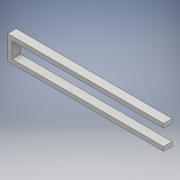
# Autodesk Inventor part: 擋車
Saved by Autodesk Inventor 2017 (Build 210142000, 142)
## iProperties
Part Number: 擋車
Material: 一般
Document SubType Name: Modeling
Designer: user
Density: 1 g/cm^3
Appearance: 預設
Author: user
Autodesk Inventor part; units mm, degrees
ref_plane "YZ Plane" through (0, 0, 0) normal (1, 0, 0) x (0, 1, 0)
ref_plane "XZ Plane" through (0, 0, 0) normal (0, 1, 0) x (-1, 0, 0)
ref_plane "XY Plane" through (0, 0, 0) normal (0, 0, 1) x (1, 0, 0)
sketch "草圖1" plane through (0, 0, 0) normal (0, 1, 0) x (-1, 0, 0)
  line L0 (-183.5, -28.5) -> (183.5, -28.5)
  line L1 (183.5, -28.5) -> (183.5, 28.5)
  line L2 (183.5, 28.5) -> (-183.5, 28.5)
  line L3 (-183.5, 28.5) -> (-183.5, -28.5)
  line L4 (-183.5, -28.5) -> (183.5, 28.5) construction
  line L5 (183.5, -28.5) -> (-183.5, 28.5) construction
  point P0 (0, 0)
  dimension "d0" = 367
  dimension "d1" = 57
  constraints: 12 end point, 2 midpoint, 2 parallel, 1 horizontal, 1 perpendicular
  measures "d0" distance of L1.end L2.end
  measures "d1" distance of L0.end L1.end
extrude "擠出1" add sketch "草圖1" along normal blind 20
sketch "草圖2" plane through (0, 20, 0) normal (0, 1, 0) x (1, 0, 0)
  line L0 (183.5, -28.5) -> (183.5, 28.5) projected
  line L1 (183.5, 18.5) -> (-173.5, 18.5)
  line L2 (-173.5, 18.5) -> (-173.5, -18.5)
  line L3 (-173.5, -18.5) -> (183.5, -18.5)
  line L4 (183.5, -18.5) -> (183.5, 18.5)
  line L5 (183.5, 28.5) -> (-183.5, 28.5) projected
  line L6 (-183.5, 28.5) -> (-183.5, -28.5) projected
  line L7 (-183.5, -28.5) -> (183.5, -28.5) projected
  point P0 (0, 0)
  dimension "d4" = 10
  dimension "d5" = 10
  dimension "d6" = 10
  constraints: 8 end point, 2 parallel, 1 horizontal, 1 perpendicular, 1 point on line
  measures "d4" distance between parallel lines of L1 L5
  measures "d5" distance between parallel lines of L6 L2
  measures "d6" distance between parallel lines of L7 L3
extrude "擠出2" cut sketch "草圖2" against normal blind 20 contours L3 L2 L1 L0
